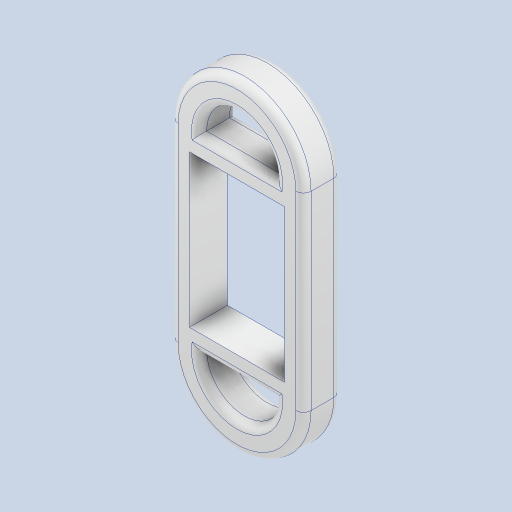
# Autodesk Inventor part: modelado
Saved by Autodesk Inventor 2024 (Build 280153000, 153)
## iProperties
Created: 2025-11-29
Part Number: modelado
Material: Aluminio 6061
Document SubType Name: Modeling
Designer: ANDRES
Density: 2.7 g/cm^3
Appearance: Aluminio - Plano
Mass: 290.227 g
Surface Area: 267.65 cm^2
Volume: 107.492 cm^3
Author: ANDRES
Autodesk Inventor part; units mm, degrees
ref_plane "YZ Plane" through (0, 0, 0) normal (1, 0, 0) x (0, 1, 0)
ref_plane "XZ Plane" through (0, 0, 0) normal (0, 1, 0) x (-1, 0, 0)
ref_plane "XY Plane" through (0, 0, 0) normal (0, 0, 1) x (1, 0, 0)
sketch "Boceto1" plane through (0, 0, 0) normal (0, 0, 1) x (1, 0, 0)
  line L0 (0, 50) -> (0, -50) construction
  line L1 (-35, 50) -> (-35, -50)
  line L2 (35, -50) -> (35, 50)
  arc A0 (35, 50) -> (-35, 50) centre (0, 50) ccw
  arc A1 (-35, -50) -> (35, -50) centre (0, -50) ccw
  line L3 (0, 11.0891) -> (0, 50) construction
  line L4 (-20, 11.0891) -> (-20, 50)
  line L5 (20, 50) -> (20, 11.0891)
  arc A2 (-20, 11.0891) -> (20, 11.0891) centre (0, 11.0891) ccw
  arc A3 (20, 50) -> (-20, 50) centre (0, 50) ccw
  line L6 (20, 50) -> (-20, 50)
  line L7 (92.9373, 0) -> (-92.9373, 0) construction
  arc A4 (-20, -50) -> (20, -50) centre (0, -50) ccw
  line L8 (20, -50) -> (-20, -50)
  line L9 (-25, 40) -> (25, 40)
  line L10 (25, 40) -> (25, -40)
  line L11 (25, -40) -> (-25, -40)
  line L12 (-25, -40) -> (-25, 40)
  line L13 (-25, 40) -> (25, -40) construction
  line L14 (25, 40) -> (-25, -40) construction
  point P0 (0, 0)
  point P1 (0, 0)
  point P2 (0, 0)
  point P3 (0, -85)
  point P4 (0, 85)
  point P5 (0, 30.5445)
  point P6 (0, 70)
  point P7 (0, 0)
  point P8 (0, 0)
  dimension "d0" = 170
  dimension "d1" = 70
  dimension "d2" = 15
  dimension "d3" = 20
  dimension "d4" = 40
  dimension "d6" = 80
  dimension "d7" = 10
  dimension "d8" = 10
  constraints: 34 end point, 13 point on circle, 8 tangent, 6 coincident, 6 midpoint, 5 centre point, 4 horizontal, 4 parallel, 3 symmetric about line, 2 vertical, 1 concentric, 1 perpendicular, 1 other
  measures "d0" distance of point (0, -85) point (0, 85)
  measures "d1" distance between parallel lines of L2 L1
  measures "d2" radial gap between concentric circles of A0 A3
  measures "d3" distance of point (0, 50) point (0, 70)
  measures "d4" distance between parallel lines of L5 L4
  measures "d6" distance between parallel lines of L11 L9
  measures "d7" distance between parallel lines of L2 L10
  measures "d8" distance between parallel lines of L8 L11
extrude "Extrusión1" add sketch "Boceto1" along normal blind 20 contours A0 L2 A1 L1 | L4 L6 L5 L9
fillet "Empalme1" radius 4 16 edges at (-35, 0, 20) (0, -85, 20) (35, 0, 20) (0, 85, 20) (0, 50, 20) (0, 70, 20) (0, -50, 20) (0, -70, 20) (0, -70, 0) (0, 85, 0) (-35, 0, 0) (0, -85, 0) (35, 0, 0) (0, 50, 0) (0, 70, 0) (0, -50, 0)
